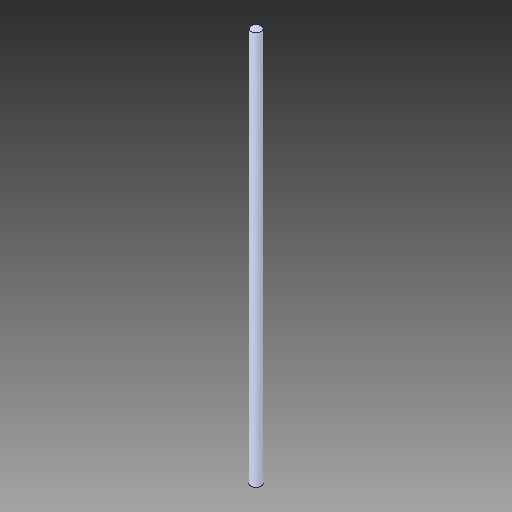
# Autodesk Inventor part: Rod1
Saved by Autodesk Inventor 2018 (Build 220112000, 112)
## iProperties
Created: 2011-02-02
Part Number: Rod1
Material: Generic
Document SubType Name: Modeling
Designer: junai
Density: 1 g/cm^3
Appearance: Default
Sending System: SolidWorks 2010
Last Author: Patrick_2
Last Saved: 2011-03-10
Author: junai
Autodesk Inventor part; units mm, degrees
ref_plane "YZ Plane" through (0, 0, 0) normal (1, 0, 0) x (0, 1, 0)
ref_plane "XZ Plane" through (0, 0, 0) normal (0, 1, 0) x (-1, 0, 0)
ref_plane "XY Plane" through (0, 0, 0) normal (0, 0, 1) x (1, 0, 0)
sketch "Sketch1" plane through (0, 0, 0) normal (0, 1, 0) x (-1, 0, 0)
  circle A0 centre (0, 0) radius 3.175
  dimension "d0" = 6.35
  constraints: 1 centre point, 1 coincident
  measures "d0" diameter of A0
extrude "Extrusion1" add sketch "Sketch1" along normal blind 250
body "Solid2"
